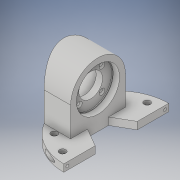
# Autodesk Inventor part: 201-
Saved by Autodesk Inventor 2018 (Build 220112000, 112)
## iProperties
Created: 2020-01-12
Part Number: 201-
Material: Generic
Document SubType Name: Modeling
Designer: Bunny320
Density: 1 g/cm^3
Appearance: Default
Author: Bunny320
Autodesk Inventor part; units mm, degrees
ref_plane "YZ Plane" through (0, 0, 0) normal (1, 0, 0) x (0, 1, 0)
ref_plane "XZ Plane" through (0, 0, 0) normal (0, 1, 0) x (-1, 0, 0)
ref_plane "XY Plane" through (0, 0, 0) normal (0, 0, 1) x (1, 0, 0)
sketch "Sketch3" plane through (0, 0, 0) normal (0, 0, 1) x (1, 0, 0)
  circle A0 centre (0, 0) radius 57.5
  dimension "d8" = 115
  constraints: 1 centre point, 1 coincident
  measures "d8" diameter of A0
extrude "Extrusion3" add sketch "Sketch3" along normal blind 8
sketch "Sketch2" plane through (0, 0, 8) normal (0, 0, 1) x (1, 0, 0)
  line L0 (-35, -30) -> (-20, -30)
  line L1 (-20, -30) -> (-20, 30)
  line L2 (-20, 30) -> (-35, 30)
  line L3 (-35, 30) -> (-35, -30)
  line L4 (-35, -30) -> (-20, 30) construction
  line L5 (-20, -30) -> (-35, 30) construction
  point P0 (0, 0)
  point P1 (-27.5, 0)
  dimension "d3" = 15
  dimension "d4" = 60
  dimension "d5" = 20
  constraints: 12 end point, 2 midpoint, 2 parallel, 1 horizontal, 1 perpendicular
  measures "d3" distance of L1.end L2.end
  measures "d4" distance of L2.end L0.start
  measures "d5" distance from line of point (0, 0) L1
extrude "Extrusion2" add sketch "Sketch2" along normal blind 62
full round fillet "Fillet1" first side at (-30, -30, 28.6667) centre faces at (-30, 10, 70) second side at (-25, 30, 49.3333)
sketch "Sketch5" plane through (0, 0, 0) normal (0, 1, 0) x (-1, 0, 0)
  line L0 (35, 215.9432) -> (32.4616, 215.9432)
  line L1 (38.0841, 40) -> (15.386, 40)
  line L2 (35, 70) -> (35, 40) projected
  line L3 (35, 53) -> (28, 53)
  line L4 (28, 53) -> (28, 63)
  line L5 (28, 63) -> (27, 63)
  line L6 (27, 63) -> (27, 63.65)
  line L7 (27, 63.65) -> (20, 63.65)
  line L8 (20, 40) -> (20, 70) projected
  point P0 (0, 0)
  point P1 (20, 42)
  dimension "d12" = 47.3
  dimension "d13" = 7
  dimension "d14" = 46
  dimension "d15" = 1
  dimension "d16" = 26
  constraints: 14 end point, 5 point on line, 4 perpendicular, 3 horizontal
  measures "d12" diameter of L7 L1
  measures "d13" distance between parallel lines of L8 L6
  measures "d14" diameter of L5 L1
  measures "d15" distance of L4.end L5.end
  measures "d16" diameter of L3 L1
revolve "Revolution1" cut sketch "Sketch5" angle 360 about axis through (-38.0841, 0, 40) along (1, 0, 0)
sketch "Sketch6" plane through (-28, 0, 40) normal (1, 0, 0) x (0, 0, -1)
  line L0 (-12.3744, -12.3744) -> (12.3744, -12.3744)
  line L1 (12.3744, -12.3744) -> (12.3744, 12.3744)
  line L2 (12.3744, 12.3744) -> (-12.3744, 12.3744)
  line L3 (-12.3744, 12.3744) -> (-12.3744, -12.3744)
  line L4 (-12.3744, -12.3744) -> (12.3744, 12.3744) construction
  line L5 (12.3744, -12.3744) -> (-12.3744, 12.3744) construction
  point P0 (40, 0)
  point P1 (0, 0)
  dimension "d17" = 35
  constraints: 12 end point, 4 coincident, 2 midpoint, 2 parallel, 2 perpendicular, 1 horizontal
  measures "d17" distance of L0.start L1.end
hole "Hole1" at (-28, 12.3744, 52.3744) at (-28, 12.3744, 27.6256) at (-28, -12.3744, 27.6256) at (-28, -12.3744, 52.3744) direction (-1, 0, 0) diameter 3.4 end through all countersink diameter 6.3 countersink angle 90 clearance for "Countersunk Flat Head Screw DIN EN ISO 2009" size "M3" standard "DIN"
sketch "Sketch7" plane through (0, 0, 8) normal (0, 0, 1) x (1, 0, 0)
  line L0 (-12.4233, 46.3644) -> (0, 0)
  line L1 (0, 80.5) -> (0, -80.5) projected
  dimension "d25" = 48
  dimension "d26" = 15
  constraints: 2 end point
  measures "d25" distance of L0.start L0.end
  measures "d26" angle of L1 L0
hole "Hole2" at (-12.4233, 46.3644, 8) direction (0, 0, -1) diameter 3.4 end through all counterbore diameter 7 counterbore depth 4 clearance for "Hex Head Cap Screw DIN EN 24017" size "M3" standard "DIN"
pattern_circular "Circular Pattern1" count 12 over 360 about axis through (0, 0, -10) along (0, 0, 1) of "Hole2" skipped copies 3 4 7 8 9 10 11 12 13 14 15 16
sketch "Sketch8" plane through (0, 0, 8) normal (0, 0, 1) x (1, 0, 0)
  line L0 (0, 23.094) -> (20, 11.547)
  line L1 (20, 11.547) -> (20, -11.547)
  line L2 (20, -11.547) -> (0, -23.094)
  line L3 (0, -23.094) -> (-20, -11.547)
  line L4 (-20, -11.547) -> (-20, 11.547)
  line L5 (-20, 11.547) -> (0, 23.094)
  point P0 (0, 0)
  point P1 (0, 0)
  dimension "d37" = 40
  constraints: 12 end point, 1 coincident, 13 other
  measures "d37" distance between parallel lines of L1 L4
extrude "Extrusion4" cut sketch "Sketch8" against normal through all
sketch "Sketch9" plane through (0, 0, 0) normal (0, 0, 1) x (1, 0, 0)
  line L0 (0, 60.5186) -> (63.6838, 60.5186)
  line L1 (63.6838, 60.5186) -> (63.6838, -58.7461)
  line L2 (63.6838, -58.7461) -> (0, -58.7461)
  line L3 (0, -58.7461) -> (0, 60.5186)
  point P0 (0, 0)
  constraints: 8 end point, 2 parallel, 1 horizontal, 1 perpendicular
extrude "Extrusion5" cut sketch "Sketch9" along normal through all
chamfer "Chamfer1" [suppressed]
fillet "Fillet3" [suppressed]
sketch "Sketch10" plane through (-35, 0, 40) normal (-1, 0, 0) x (0, 0, 1)
  line L0 (-40, 57.5) -> (-40, -57.5) projected
  line L1 (-40, -57.5) -> (-32, -57.5) projected
  line L2 (-32, 57.5) -> (-40, 57.5) projected
  line L3 (-33.25, 51.9123) -> (-36, 50.3246)
  line L4 (-36, 50.3246) -> (-38.75, 51.9123)
  line L5 (-38.75, 51.9123) -> (-38.75, 55.0877)
  line L6 (-38.75, 55.0877) -> (-36, 56.6754)
  line L7 (-36, 56.6754) -> (-33.25, 55.0877)
  line L8 (-33.25, 55.0877) -> (-33.25, 51.9123)
  point P0 (-40, 0)
  point P1 (-36, 53.5)
  point P2 (-36, -53.5)
  point P3 (-36, 53.5)
  dimension "d55" = 4
  dimension "d56" = 4
  dimension "d57" = 4
  dimension "d58" = 4
  dimension "d67" = 5.5
  constraints: 12 end point, 1 coincident, 1 vertical, 13 other
  measures "d55" distance from line of L0 point (-36, -53.5)
  measures "d56" distance from line of L1 point (-36, -53.5)
  measures "d57" distance from line of L2 point (-36, 53.5)
  measures "d58" distance from line of L0 point (-36, 53.5)
  measures "d67" distance between parallel lines of L5 L8
hole "Hole4" at (-35, -53.5, 4) direction (1, 0, 0) diameter 3.4 end through all counterbore diameter 6 counterbore depth 30 clearance for "Hex Head Cap Screw DIN EN 24017" size "M3" standard "DIN"
hole "Hole5" at (-35, 53.5, 4) direction (1, 0, 0) diameter 3.4 end through all clearance for "Countersunk Flat Head Screw DIN EN ISO 2009" size "M3" standard "DIN"
extrude "Extrusion6" cut sketch "Sketch10" against normal blind 30
sketch "Sketch12" plane through (-35, -30, 8) normal (-1, 0, 0) x (0, 0, 1)
  circle A0 centre (32, 30) radius 13 projected
  circle A1 centre (32, 30) radius 21.1
  arc A2 (32, 0) -> (32, 60) centre (32, 30) ccw projected
  line L0 (0, 0) -> (32, 0) projected
  line L1 (0, 60) -> (32, 60) projected
  line L2 (0, 0) -> (0, 60) projected
  point P0 (-8, 30)
  dimension "d79" = 42.2
  constraints: 1 centre point, 1 coincident
  measures "d79" diameter of A1
extrude "Extrusion7" add sketch "Sketch12" along normal up to surface contours L0 L2 L1 A2 round surface about axis through (0, 0, 0) along (0, 0, 1) radius 57.5 far side no
equation "\"d55\" = 0.5 * d9"
equation "\"d56\" = 0.5 * d9"
equation "\"d57\" = 0.5 * d9"
equation "\"d58\" = 0.5 * d9"
equation "\"d9\" = 8"
body "Solid1"
